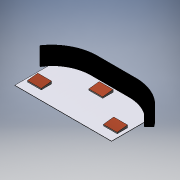
# Autodesk Inventor part: Charging Dock
Saved by Autodesk Inventor 2018 (Build 220112000, 112)
## iProperties
Created: 2017-03-09
Part Number: Charging Dock
Material: ABS Plastic
Document SubType Name: Modeling
Designer: Eightfold_Infotech
Density: 1.06 g/cm^3
Appearance: Smooth - White
Author: Eightfold_Infotech
Autodesk Inventor part; units mm, degrees
ref_plane "YZ Plane" through (0, 0, 0) normal (1, 0, 0) x (0, 1, 0)
ref_plane "XZ Plane" through (0, 0, 0) normal (0, 1, 0) x (-1, 0, 0)
ref_plane "XY Plane" through (0, 0, 0) normal (0, 0, 1) x (1, 0, 0)
sketch "Sketch1" plane through (0, 0, 0) normal (0, 1, 0) x (-1, 0, 0)
  line L0 (-50, -122.5) -> (50, -122.5)
  line L1 (50, -122.5) -> (50, -47.5)
  line L2 (50, -47.5) -> (-50, -47.5)
  line L3 (-50, -47.5) -> (-50, -122.5)
  line L4 (-50, -122.5) -> (50, -47.5) construction
  line L5 (50, -122.5) -> (-50, -47.5) construction
  line L6 (-325, 122.5) -> (-225, 122.5)
  line L7 (-225, 122.5) -> (-225, 47.5)
  line L8 (-225, 47.5) -> (-325, 47.5)
  line L9 (-325, 47.5) -> (-325, 122.5)
  line L10 (-325, 122.5) -> (-225, 47.5) construction
  line L11 (-225, 122.5) -> (-325, 47.5) construction
  line L12 (0, 214.4175) -> (0, -235.835)
  line L13 (325, 122.5) -> (225, 122.5)
  line L14 (225, 122.5) -> (225, 47.5)
  line L15 (225, 47.5) -> (325, 47.5)
  line L16 (325, 47.5) -> (325, 122.5)
  line L17 (325, 122.5) -> (225, 47.5) construction
  line L18 (225, 122.5) -> (325, 47.5) construction
  point P0 (0, 0)
  point P1 (0, -85)
  point P2 (-275, 85)
  point P3 (275, 85)
  dimension "d0" = 100
  dimension "d1" = 75
  dimension "d2" = 85
  dimension "d3" = 100
  dimension "d4" = 75
  dimension "d5" = 275
  dimension "d6" = 85
  constraints: 38 end point, 6 midpoint, 5 symmetric about line, 4 parallel, 2 horizontal, 2 perpendicular, 1 vertical
  measures "d0" distance of L2.end L1.end
  measures "d1" distance of L1.end L0.end
  measures "d2" distance of point (0, 0) point (0, -85)
  measures "d3" distance of L7.end L8.end
  measures "d4" distance of L6.end L7.end
  measures "d5" horizontal distance of point (0, 0) point (-275, 85)
  measures "d6" vertical distance of point (0, 0) point (-275, 85)
sketch "Sketch2" plane through (0, 0, 0) normal (0, 1, 0) x (-1, 0, 0)
  line L0 (-7.5, -95) -> (7.5, -95) projected
  line L1 (7.5, -95) -> (7.5, -75) projected
  line L2 (7.5, -75) -> (-7.5, -75) projected
  line L3 (-7.5, -75) -> (-7.5, -95) projected
  line L4 (267.5, 95) -> (267.5, 75) projected
  line L5 (267.5, 75) -> (282.5, 75) projected
  line L6 (282.5, 75) -> (282.5, 95) projected
  line L7 (282.5, 95) -> (267.5, 95) projected
  line L8 (-267.5, 95) -> (-282.5, 95) projected
  line L9 (-282.5, 95) -> (-282.5, 75) projected
  line L10 (-282.5, 75) -> (-267.5, 75) projected
  line L11 (-267.5, 75) -> (-267.5, 95) projected
  line L12 (-137.5, -150) -> (137.5, -150)
  line L13 (137.5, -150) -> (137.5, -200)
  line L14 (137.5, -200) -> (-137.5, -200)
  line L15 (-137.5, -200) -> (-137.5, -150)
  line L16 (-137.5, -150) -> (137.5, -200) construction
  line L17 (137.5, -150) -> (-137.5, -200) construction
  arc A0 (-376.4677, -20.0539) -> (-137.5, -150) centre (-137.5, 134.7009) ccw
  line L18 (-137.5, -150) -> (-137.5, 134.7009) construction
  line L19 (-412.5, 61.0149) -> (-137.5, 134.7009) construction
  arc A1 (-412.5, -56.0862) -> (-137.5, -200) centre (-137.5, 134.7009) ccw
  line L20 (0, -269.3547) -> (0, -73.2831)
  arc A2 (137.5, -150) -> (376.4677, -20.0539) centre (137.5, 134.7009) ccw
  arc A3 (137.5, -200) -> (412.5, -56.0862) centre (137.5, 134.7009) ccw
  line L21 (412.5, -56.0862) -> (376.4677, -20.0539)
  line L22 (412.5, -56.0862) -> (463.4573, -56.0862) construction
  line L23 (-412.5, -56.0862) -> (-376.4677, -20.0539)
  point P0 (0, 0)
  point P1 (0, -175)
  point P2 (412.5, 61.0149)
  dimension "d9" = 275
  dimension "d10" = 50
  dimension "d11" = 100
  dimension "d12" = 75
  dimension "d17" = 135
  constraints: 24 end point, 8 point on circle, 5 symmetric about line, 4 centre point, 2 coincident, 2 horizontal, 2 midpoint, 2 parallel, 1 equal length, 1 perpendicular, 1 tangent, 1 vertical, 2 other
  measures "d9" distance of L13.end L14.end
  measures "d10" distance of L12.end L13.end
  measures "d11" distance from line of L2 point (0, -175)
  measures "d12" angle of L19 L18
  measures "d17" angle of L22 L21
extrude "Extrusion2" add sketch "Sketch2" along normal blind 100 contours L12 L13 L14 L20 | L20 L14 L15 L12 | L15 A1 L23 A0 | A2 L21 A3 L13
fillet "Fillet1" radius 3 12 edges at (0, 100, -150) (273.507, 100, -115.4125) (-273.507, 100, -115.4125) (-394.4839, 100, -38.07) (394.4839, 100, -38.07) (-376.4677, 50, -20.0539) (-412.5, 50, -56.0862) (376.4677, 50, -20.0539) (412.5, 50, -56.0862) (-292.6904, 100, -161.847) (292.6904, 100, -161.847) (0, 100, -200)
sketch "Sketch3" plane through (0, 0, 0) normal (0, -1, 0) x (1, 0, 0)
  line L0 (350, 188.4615) -> (-350, 188.4615)
  line L1 (-350, 188.4615) -> (-350, -54.7677)
  line L2 (350, -54.7677) -> (350, 188.4615)
  arc A0 (411.0516, -58.1571) -> (410.721, -54.3072) centre (408.5997, -56.4285) ccw projected
  line L3 (379.0735, -22.6597) -> (410.721, -54.3072) projected
  arc A1 (379.0735, -22.6597) -> (374.4553, -23.118) centre (376.9522, -24.781) ccw projected
  arc A2 (137.5, -150) -> (374.4553, -23.118) centre (137.5, 134.7009) ccw projected
  line L4 (-137.5, -150) -> (137.5, -150) projected
  arc A3 (-374.4553, -23.118) -> (-137.5, -150) centre (-137.5, 134.7009) ccw projected
  arc A4 (-374.4553, -23.118) -> (-379.0735, -22.6597) centre (-376.9522, -24.781) ccw projected
  line L5 (-410.721, -54.3072) -> (-379.0735, -22.6597) projected
  arc A5 (-410.721, -54.3072) -> (-411.0516, -58.1571) centre (-408.5997, -56.4285) ccw projected
  arc A6 (-411.0516, -58.1571) -> (-137.5, -200) centre (-137.5, 134.7009) ccw projected
  line L6 (137.5, -200) -> (-137.5, -200) projected
  arc A7 (137.5, -200) -> (411.0516, -58.1571) centre (137.5, 134.7009) ccw projected
  arc A8 (137.5, -200) -> (411.0516, -58.1571) centre (137.5, 134.7009) ccw projected
  line L7 (0, -256.7037) -> (0, -18.0297)
  point P0 (0, 0)
  dimension "d31" = 700
  constraints: 8 end point, 3 point on circle, 1 horizontal, 1 parallel, 1 perpendicular, 1 vertical
  measures "d31" distance of L0.start L0.end
extrude "Extrusion3" add sketch "Sketch3" against normal blind 2 contours L2 A2 L4 A3 L1 L0
extrude "Extrusion6" add sketch "Sketch1" along normal blind 20
sketch "Sketch6" plane through (325, 2, 47.5) normal (1, 0, 0) x (0, 0, -1)
  line L0 (0, 0) -> (-75, 0) projected
  line L1 (0, 0) -> (0, 18) projected
  line L2 (-75, 18) -> (0, 18) projected
  line L3 (-75, 0) -> (-75, 18) projected
  line L4 (0, 0) -> (0, 18) projected
  line L5 (0, 18) -> (-75, 9)
  line L6 (-75, 0) -> (-75, 18) projected
  line L7 (-75, 18) -> (0, 18)
  line L8 (-75, 9) -> (-75, 18)
  point P0 (47.5, -2)
  constraints: 6 end point, 1 collinear, 1 midpoint, 1 perpendicular
extrude "Extrusion7" cut sketch "Sketch6" against normal through all contours L5 L3 L2
sketch "Sketch7" plane through (50, 2, -122.5) normal (1, 0, 0) x (0, 0, -1)
  line L0 (0, 0) -> (-75, 0) projected
  line L1 (0, 0) -> (0, 18) projected
  line L2 (-75, 18) -> (0, 18) projected
  line L3 (-75, 0) -> (-75, 18) projected
  line L4 (0, 18) -> (-75, 9)
  line L5 (-75, 9) -> (-75, 18)
  line L6 (-75, 18) -> (0, 18) projected
  line L7 (-75, 18) -> (0, 18)
  point P0 (-122.5, -2)
  constraints: 6 end point, 1 collinear, 1 horizontal, 1 midpoint
extrude "Extrusion8" cut sketch "Sketch7" against normal up to surface (100 mm away) contours L4 L3 L2
body "Solid1"
